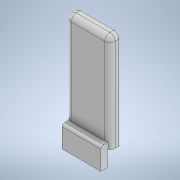
# Autodesk Inventor part: BluetoothModule
Saved by Autodesk Inventor 2020 (Build 240168000, 168)
## iProperties
Created: 2020-04-08
Part Number: BluetoothModule
Material: Generic
Document SubType Name: Modeling
Designer: Samuele
Density: 1 g/cm^3
Appearance: Default
Author: Samuele
Autodesk Inventor part; units mm, degrees
ref_plane "YZ Plane" through (0, 0, 0) normal (1, 0, 0) x (0, 1, 0)
ref_plane "XZ Plane" through (0, 0, 0) normal (0, 1, 0) x (-1, 0, 0)
ref_plane "XY Plane" through (0, 0, 0) normal (0, 0, 1) x (1, 0, 0)
sketch "Sketch1" plane through (0, 0, 0) normal (0, 0, 1) x (1, 0, 0)
  line L0 (0, 0) -> (17, 0)
  line L1 (17, 0) -> (17, 38)
  line L2 (17, 38) -> (0, 38)
  line L3 (0, 38) -> (0, 0)
  dimension "d0" = 17
  dimension "d1" = 38
  constraints: 8 end point, 2 parallel, 1 horizontal, 1 perpendicular
  measures "d0" distance of L2.end L1.end
  measures "d1" distance of L1.end L0.end
extrude "Extrusion1" add sketch "Sketch1" along normal blind 4
fillet "Fillet1" radius 2 5 edges at (17, 19, 4) (0, 19, 4) (8.5, 38, 4) (17, 38, 2) (0, 38, 2)
fillet "Fillet2" radius 0.5 5 edges at (0.5858, 37.4142, 0) (8.5, 38, 0) (16.4142, 37.4142, 0) (17, 18, 0) (0, 18, 0)
sketch "Sketch2" plane through (0, 0, 2) normal (-1, 0, 0) x (0, 0, 1)
  line L0 (2, 0) -> (4.5, 0)
  line L1 (4.5, 0) -> (4.5, -6)
  line L2 (4.5, -6) -> (2, -6)
  line L3 (2, -6) -> (2, 0)
  line L4 (4.5, 0) -> (4.5, 2.5)
  line L5 (4.5, 2.5) -> (2, 2.5)
  line L6 (2, 2.5) -> (-2, 2.5)
  line L7 (-2, 36) -> (-2, 0) projected
  line L8 (-2, 2.5) -> (-2, 0)
  line L9 (2, 0) -> (0, 0) projected
  line L10 (-2, 0) -> (2, 0)
  dimension "d6" = 2.5
  dimension "d7" = 6
  dimension "d8" = 2.5
  dimension "d9" = 2.5
  constraints: 18 end point, 3 horizontal, 3 perpendicular, 2 vertical, 1 point on line
  measures "d6" distance of L0.start L0.end
  measures "d7" distance of L0.end L1.end
  measures "d8" distance of L1.end L2.end
  measures "d9" distance of L0.end L4.end
extrude "Extrusion2" add sketch "Sketch2" against normal blind 16
fillet "Fillet3" radius 0.5 1 edges at (0, 1.25, 0)
sketch "Sketch3" plane through (0, 0, 0.5) normal (-1, 0, 0) x (0, 0, 1)
  line L0 (3.5, 0) -> (3.5, -6) projected
  line L1 (6, -6) -> (6, 2.5) projected
  line L2 (3.5, -6) -> (6, -6)
  line L3 (6, -6) -> (6, 2.5)
  line L4 (6, 2.5) -> (3.5, 2.5)
  line L5 (3.5, 2.5) -> (3.5, -6)
  point P0 (-0.5, 0)
  constraints: 8 end point, 2 parallel, 1 horizontal, 1 perpendicular
extrude "Extrusion3" cut sketch "Sketch3" against normal blind 1
fillet "Fillet4" radius 2.5 1 edges at (0, 1.25, 4)
fillet "Fillet5" radius 1 1 edges at (8.5, 2.5, 6.5)
body "Solid1"
